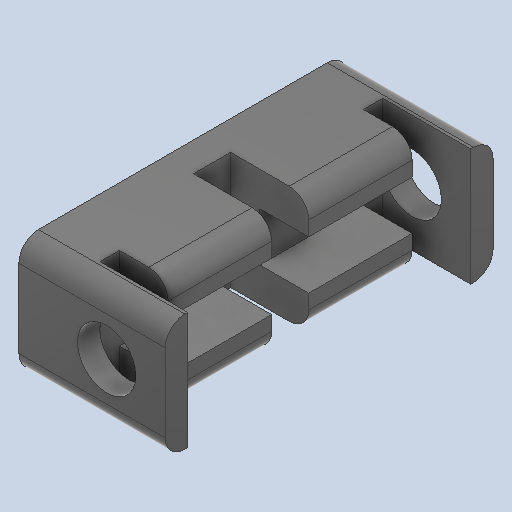
# Autodesk Inventor part: Cable_fixing
Saved by Autodesk Inventor 2022.4 (Build 264492000, 492)
## iProperties
Created: 2021-09-09
Part Number: Cable_fixing
Material: 熱可塑性 樹脂
Document SubType Name: Modeling
Designer: Hiroki Noguchi
Density: 1.28 g/cm^3
Appearance: 滑らか - 黒
Description: TPU
Mass: 4.22814 g
Surface Area: 23.5358 cm^2
Volume: 3.30324 cm^3
Author: Hiroki Noguchi
Autodesk Inventor part; units mm, degrees
ref_plane "YZ Plane" through (0, 0, 0) normal (1, 0, 0) x (0, 1, 0)
ref_plane "XZ Plane" through (0, 0, 0) normal (0, 1, 0) x (-1, 0, 0)
ref_plane "XY Plane" through (0, 0, 0) normal (0, 0, 1) x (1, 0, 0)
sketch "スケッチ1" plane through (0, 0, 0) normal (0, 0, 1) x (1, 0, 0)
  line L0 (7.5, -6) -> (-7.5, -6)
  line L1 (-7.5, -6) -> (-7.5, 6)
  line L2 (-7.5, 6) -> (7.5, 6)
  line L3 (7.5, 6) -> (7.5, -6)
  line L4 (7.5, -6) -> (-7.5, 6) construction
  line L5 (-7.5, -6) -> (7.5, 6) construction
  point P0 (0, 0)
  point P1 (0, 0)
  point P2 (0, 0)
  dimension "d2" = 15
  dimension "d4" = 12
  constraints: 12 end point, 3 midpoint, 2 parallel, 1 coincident, 1 horizontal, 1 perpendicular
  measures "d2" distance of L1.end L2.end
  measures "d4" distance between parallel lines of L0 L2
extrude "押し出し1" add sketch "スケッチ1" along normal mid plane 33.6
sketch "スケッチ3" plane through (7.5, -6, -16.8) normal (1, 0, 0) x (0, 0, -1)
  line L0 (-29.3, 8.5) -> (-4.3, 8.5)
  line L1 (-4.3, 8.5) -> (-4.3, 3.5)
  line L2 (-4.3, 3.5) -> (-29.3, 3.5)
  line L3 (-29.3, 3.5) -> (-29.3, 8.5)
  line L4 (-29.3, 8.5) -> (-4.3, 3.5) construction
  line L5 (-4.3, 8.5) -> (-29.3, 3.5) construction
  line L6 (-31.3, 12) -> (-29.3, 12)
  line L7 (-29.3, 12) -> (-29.3, 0)
  line L8 (-29.3, 0) -> (-31.3, 0)
  line L9 (-31.3, 0) -> (-31.3, 12)
  line L10 (0, 0) -> (-33.6, 0) projected
  line L11 (-2.3, 12) -> (-2.3, 0)
  line L12 (-4.3, 0) -> (-4.3, 12)
  line L13 (-2.3, 0) -> (-4.3, 0)
  line L14 (-4.3, 12) -> (-2.3, 12)
  point P0 (-16.8, 6)
  point P1 (-16.8, 6)
  point P2 (-16.8, 6)
  point P3 (-29.3, 6)
  point P4 (-30.3, 0)
  point P5 (-18.35, 0)
  point P6 (-4.3, 6)
  point P7 (-3.3, 12)
  point P8 (-4.3, 3.5)
  dimension "d11" = 25
  dimension "d14" = 12
  dimension "d15" = 2
  dimension "d18" = 360
  dimension "d26" = 5
  constraints: 28 end point, 7 midpoint, 4 parallel, 2 horizontal, 2 perpendicular, 1 coincident, 1 point on line, 21 other
  measures "d11" distance between parallel lines of L1 L3
  measures "d14" distance between parallel lines of L8 L6
  measures "d15" distance between parallel lines of L9 L7
  measures "d26" distance between parallel lines of L2 L0
extrude "押し出し3" cut sketch "スケッチ3" against normal blind 9 contours L0 L1 L2 L3 | L3 L7 L8 L9 L6 | L12 L14 L11 L10 L1
sketch "スケッチ4" plane through (0, 0, -16.8) normal (0, 0, -1) x (-1, 0, 0)
  circle A0 centre (-1.5, 0) radius 3
  line L0 (-7.5, 6) -> (-7.5, -6) projected
  point P0 (0, 0)
  dimension "d22" = 6
  dimension "d23" = 6
  constraints: 1 centre point, 1 horizontal alignment
  measures "d22" diameter of A0
  measures "d23" distance from line of L0 A0.centre
extrude "押し出し4" cut sketch "スケッチ4" against normal up to surface (2.3 mm away)
mirror "ミラー1" about plane through (0, 0, 0) normal (0, 0, 1) of "押し出し4"
sketch "スケッチ5" plane through (-7.5, 6, -16.8) normal (0, 1, 0) x (1, 0, 0)
  line L0 (15, -4.3) -> (15, -29.3) projected
  line L1 (6, -4.3) -> (15, -4.3) projected
  line L2 (15, -29.3) -> (11, -29.3)
  line L3 (11, -29.3) -> (11, -4.3)
  line L4 (11, -4.3) -> (15, -4.3)
  line L5 (15, -4.3) -> (15, -29.3)
  line L6 (11, -18.7) -> (3, -18.7)
  line L7 (3, -18.7) -> (3, -14.9)
  line L8 (3, -14.9) -> (11, -14.9)
  line L9 (11, -14.9) -> (11, -18.7)
  point P0 (11, -16.8)
  point P1 (11, -16.8)
  dimension "d30" = 4
  dimension "d36" = 8
  dimension "d37" = 3.8
  constraints: 16 end point, 4 parallel, 2 coincident, 2 horizontal, 2 midpoint, 2 perpendicular, 1 point on line
  measures "d30" distance of L3.end L4.end
  measures "d36" distance of L7.end L8.end
  measures "d37" distance of L6.end L7.end
extrude "押し出し5" cut sketch "スケッチ5" against normal through all
fillet "フィレット4" radius 2 8 edges at (0, 6, -16.8) (0, -6, -16.8) (0, 6, 16.8) (0, -6, 16.8) (3.5, 6, 7.2) (3.5, 6, -7.2) (3.5, -6, -7.2) (3.5, -6, 7.2)
